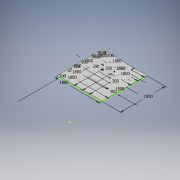
# Autodesk Inventor part: Bodenplatte_korrigiert
Saved by Autodesk Inventor 2019 (Build 230136000, 136)
## iProperties
Created: 2021-09-26
Part Number: Bodenplatte_korrigiert
Material: Generisch
Document SubType Name: Modeling
Designer: mritt
Density: 1 g/cm^3
Appearance: Vorgabe
Author: mritt
Autodesk Inventor part; units mm, degrees
ref_plane "YZ Plane" through (0, 0, 0) normal (1, 0, 0) x (0, 1, 0)
ref_plane "XZ Plane" through (0, 0, 0) normal (0, 1, 0) x (-1, 0, 0)
ref_plane "XY Plane" through (0, 0, 0) normal (0, 0, 1) x (1, 0, 0)
sketch "Skizze1" plane through (0, 0, 0) normal (0, 1, 0) x (-1, 0, 0)
  line L0 (1866.4377, -1385.0115) -> (66.4377, -1385.0115)
  line L1 (66.4377, -1385.0115) -> (66.4377, -3185.0115)
  line L2 (366.4377, -1385.0115) -> (366.4377, -3185.0115)
  line L3 (666.4377, -3185.0115) -> (666.4377, -1385.0115)
  line L4 (966.4377, -1385.0115) -> (966.4377, -3185.0115)
  line L5 (1266.4377, -3185.0115) -> (1266.4377, -1385.0115)
  line L6 (1566.4377, -1385.0115) -> (1566.4377, -3185.0115)
  line L7 (66.4377, -1685.0115) -> (1866.4377, -1685.0115)
  line L8 (66.4377, -1985.0115) -> (1866.4377, -1985.0115)
  line L9 (66.4377, -2285.0115) -> (1866.4377, -2285.0115)
  line L10 (66.4377, -2585.0115) -> (1866.4377, -2585.0115)
  line L11 (66.4377, -2885.0115) -> (1866.4377, -2885.0115)
  line L12 (66.4377, -3185.0115) -> (1866.4377, -3185.0115)
  line L13 (1866.4377, -1385.0115) -> (1866.4377, -3185.0115)
  point P0 (0, 0)
  point P1 (1870.1754, -1685.0115)
  point P2 (1566.4377, -1685.0115)
  point P3 (1266.4377, -1685.0115)
  point P4 (966.4377, -1685.0115)
  point P5 (666.4377, -1685.0115)
  point P6 (366.4377, -1685.0115)
  point P7 (366.4377, -1985.0115)
  point P8 (666.4377, -1985.0115)
  point P9 (966.4377, -1985.0115)
  point P10 (1266.4377, -1985.0115)
  point P11 (1566.4377, -1985.0115)
  point P12 (1870.1754, -1985.0115)
  point P13 (1870.1754, -2285.0115)
  point P14 (1566.4377, -2285.0115)
  point P15 (1266.4377, -2285.0115)
  point P16 (966.4377, -2285.0115)
  point P17 (666.4377, -2285.0115)
  point P18 (366.4377, -2285.0115)
  point P19 (366.4377, -2585.0115)
  point P20 (666.4377, -2585.0115)
  point P21 (966.4377, -2585.0115)
  point P22 (1266.4377, -2585.0115)
  point P23 (1566.4377, -2585.0115)
  point P24 (1870.1754, -2585.0115)
  point P25 (1870.1754, -2885.0115)
  point P26 (1566.4377, -2885.0115)
  point P27 (1266.4377, -3185.0115)
  point P28 (1266.4377, -2885.0115)
  point P29 (966.4377, -2885.0115)
  point P30 (966.4377, -3185.0115)
  point P31 (666.4377, -3185.0115)
  point P32 (666.4377, -2885.0115)
  point P33 (366.4377, -2885.0115)
  point P34 (366.4377, -3185.0115)
  point P35 (1866.4377, -3185.0115)
  dimension "d0" = 1800
  dimension "d2" = 300
  dimension "d3" = 300
  dimension "d4" = 300
  dimension "d5" = 300
  dimension "d6" = 300
  dimension "d8" = 300
  dimension "d9" = 300
  dimension "d10" = 300
  dimension "d11" = 300
  dimension "d12" = 300
  dimension "d32" = 1800
  dimension "d33" = 1800
  dimension "d34" = 1800
  dimension "d35" = 1800
  dimension "d36" = 1800
  dimension "d37" = 1800
  dimension "d38" = 1800
  dimension "d39" = 1800
  dimension "d40" = 1800
  dimension "d41" = 1800
  dimension "d42" = 1800
  dimension "d43" = 1800
  dimension "d44" = 300
  dimension "d45" = 300
  constraints: 62 point on line, 28 end point, 12 midpoint, 3 perpendicular, 1 horizontal
  measures "d0" distance of L0.end L1.end
  measures "d2" distance between parallel lines of L2 L1
  measures "d3" distance between parallel lines of L2 L3
  measures "d4" distance between parallel lines of L3 L4
  measures "d5" distance between parallel lines of L4 L5
  measures "d6" distance between parallel lines of L5 L6
  measures "d8" distance between parallel lines of L7 L0
  measures "d9" distance between parallel lines of L8 L7
  measures "d10" distance between parallel lines of L8 L9
  measures "d11" distance between parallel lines of L10 L9
  measures "d12" distance between parallel lines of L11 L10
  measures "d32" distance of L3.start L3.end
  measures "d33" distance of L4.start L4.end
  measures "d34" distance of L5.start L5.end
  measures "d35" distance of L6.start L6.end
  measures "d36" distance of L13.start L13.end
  measures "d37" distance of L12.start L12.end
  measures "d38" distance of L11.start L11.end
  measures "d39" distance of L10.start L10.end
  measures "d40" distance of L9.start L9.end
  measures "d41" distance of L8.start L8.end
  measures "d42" distance of L7.start L7.end
  measures "d43" distance of L0.start L0.end
  measures "d44" distance between parallel lines of L6 L13
  measures "d45" distance between parallel lines of L12 L11
extrude "Extrusion3" add sketch "Skizze1" along normal blind 20
hole "Bohrung3" at (-1870.1754, 0, -1685.0115) at (-1566.4377, 0, -1685.0115) at (-1266.4377, 0, -1685.0115) at (-966.4377, 0, -1685.0115) at (-666.4377, 0, -1685.0115) at (-366.4377, 0, -1685.0115) at (-366.4377, 0, -1985.0115) at (-666.4377, 0, -1985.0115) at (-966.4377, 0, -1985.0115) at (-1266.4377, 0, -1985.0115) at (-1566.4377, 0, -1985.0115) at (-1870.1754, 0, -1985.0115) at (-1870.1754, 0, -2285.0115) at (-1566.4377, 0, -2285.0115) at (-1266.4377, 0, -2285.0115) at (-966.4377, 0, -2285.0115) at (-666.4377, 0, -2285.0115) at (-366.4377, 0, -2285.0115) at (-366.4377, 0, -2585.0115) at (-666.4377, 0, -2585.0115) at (-966.4377, 0, -2585.0115) at (-1266.4377, 0, -2585.0115) at (-1566.4377, 0, -2585.0115) at (-1870.1754, 0, -2585.0115) at (-1870.1754, 0, -2885.0115) at (-1566.4377, 0, -2885.0115) at (-1566.4377, 0, -3185.0115) at (-1266.4377, 0, -3185.0115) at (-1266.4377, 0, -2885.0115) at (-966.4377, 0, -2885.0115) at (-966.4377, 0, -3185.0115) at (-666.4377, 0, -3185.0115) at (-666.4377, 0, -2885.0115) at (-366.4377, 0, -2885.0115) at (-366.4377, 0, -3185.0115) at (-1866.4377, 0, -3185.0115) direction (0, 1, 0) diameter 9.376 end through all thread size "M11x1.5" class "6H" standard "ANSI Metric M Profile"
